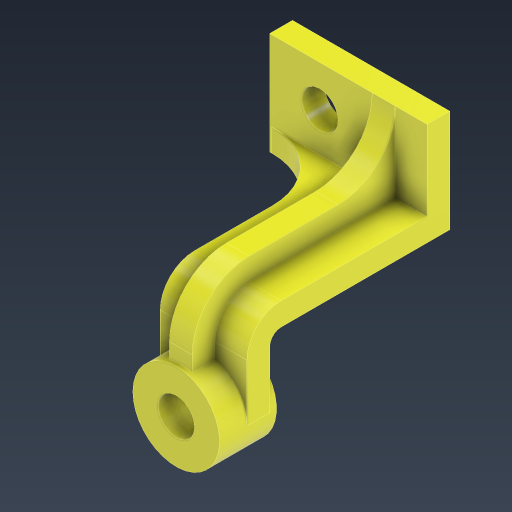
# Autodesk Inventor part: Peça teste
Saved by Autodesk Inventor 2024 (Build 280153000, 153)
## iProperties
Created: 2024-02-09
Part Number: Peça teste
Material: Genérico
Document SubType Name: Modeling
Designer: Administrator
Density: 1 g/cm^3
Appearance: Amarelo
Author: Administrator
Autodesk Inventor part; units mm, degrees
ref_plane "YZ Plane" through (0, 0, 0) normal (1, 0, 0) x (0, 1, 0)
ref_plane "XZ Plane" through (0, 0, 0) normal (0, 1, 0) x (-1, 0, 0)
sketch "Esboço1" plane through (0, 0, 0) normal (0, 0, 1) x (1, 0, 0)
  line L0 (0, 0) -> (69, 0)
  line L1 (69, 0) -> (69, 45)
  line L2 (69, 45) -> (0, 45)
  line L3 (0, 45) -> (0, 0)
  dimension "d0" = 69
  dimension "d1" = 45
  constraints: 8 end point, 2 parallel, 1 horizontal, 1 perpendicular
  measures "d0" distance of L2.end L1.end
  measures "d1" distance of L1.end L0.end
extrude "Extrusão1" add sketch "Esboço1" along normal mid plane 10
ref_plane "Plano de trabalho1" through (0, 0, 96) normal (0, 0, -1) x (-1, 0, 0)
sketch "Esboço3" plane through (0, 0, 96) normal (0, 0, -1) x (-1, 0, 0)
  circle A0 centre (-50, -30) radius 19
  line L0 (-69, 0) -> (-69, 45) projected
  line L1 (-69, 45) -> (0, 45) projected
  point P0 (0, 0)
  dimension "d8" = 38
  dimension "d9" = 75
  constraints: 1 centre point, 1 tangent
  measures "d8" diameter of A0
  measures "d9" distance from line of A0.centre L1
extrude "Extrusão3" add sketch "Esboço3" along normal blind 25
sketch "Esboço4" plane through (69, 0, 5) normal (1, 0, 0) x (0, 0, -1)
  line L0 (0, 45) -> (0, 0) construction
  line L1 (0, 0) -> (-64, 0)
  line L2 (-69, -5) -> (-69, -30)
  line L3 (-69, -30) -> (-79, -30)
  line L4 (-79, -30) -> (-79, -5)
  line L5 (-64, 10) -> (0, 10)
  line L6 (-91, -49) -> (-91, -11) construction
  line L7 (-91, -30) -> (-66, -30) construction
  line L8 (-66, -49) -> (-66, -11) construction
  arc A0 (-64, 0) -> (-69, -5) centre (-64, -5) ccw
  arc A1 (-64, 10) -> (-79, -5) centre (-64, -5) ccw
  point P0 (5, 0)
  dimension "d12" = 10
  dimension "d13" = 10
  dimension "d14" = 3
  dimension "d15" = 5
  dimension "d16" = 15
  constraints: 12 end point, 4 perpendicular, 4 point on circle, 4 tangent, 2 centre point, 2 midpoint, 2 point on line, 1 horizontal
  measures "d12" distance between parallel lines of L1 L5
  measures "d13" distance between parallel lines of L4 L2
  measures "d14" distance between parallel lines of L8 L2
  measures "d15" radius of A0
  measures "d16" radius of A1
extrude "Extrusão4" add sketch "Esboço4" against normal blind 38 fills toward (-32, 0.05) open curves L1 A0 L2 L3 L4 A1 L5
sketch "Esboço5" plane through (0, 0, 5) normal (0, 0, 1) x (1, 0, 0)
  line L0 (69, 10) -> (31, 10) projected
  line L1 (45, 10) -> (55, 10)
  line L2 (55, 10) -> (55, 20)
  line L3 (55, 20) -> (45, 20)
  line L4 (45, 20) -> (45, 10)
  line L5 (31, 10) -> (31, -5) projected
  point P0 (0, 0)
  dimension "d20" = 10
  dimension "d21" = 10
  dimension "d22" = 14
  constraints: 8 end point, 2 parallel, 1 horizontal, 1 perpendicular, 1 point on line
  measures "d20" distance of L3.end L2.end
  measures "d21" distance of L2.end L1.end
  measures "d22" distance between parallel lines of L5 L4
sketch3d "Esboço 3D1"
  line L0 (69, 10, 5) -> (69, 10, 69)
  arc A0 (69, 10, 69) -> (69, -5, 84) centre (69, -5, 69) ccw
  line L1 (69, -5, 84) -> (69, -30, 84)
sweep "Varredura1" add profiles "Esboço5" path "Esboço 3D1"
fillet "Arredondamento1" radius 25 1 edges at (50, 20, 5)
fillet "Arredondamento2" radius 30 1 edges at (31, 5, 5)
sketch "Esboço6" plane through (50, -30, 96) normal (0, 0, 1) x (1, 0, 0)
  circle A0 centre (0, 0) radius 19 projected
  point P0 (-50, 30)
  constraints: 1 coincident
hole "Furo1" at (50, -30, 96) direction (0, 0, -1) diameter 16 end through all
sketch "Esboço7" plane through (0, 0, 5) normal (0, 0, 1) x (1, 0, 0)
  line L0 (45, 45) -> (0, 45) projected
  line L1 (0, 45) -> (0, 0) projected
  point P0 (22, 27)
  dimension "d34" = 18
  dimension "d35" = 22
  measures "d34" distance from line of L0 point (22, 27)
  measures "d35" distance from line of L1 point (22, 27)
hole "Furo2" at (22, 27, 5) direction (0, 0, -1) diameter 16 end through all
